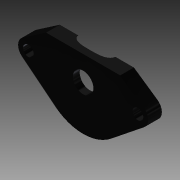
# Autodesk Inventor part: Bearing Cover
Saved by Autodesk Inventor 2013 (Build 170138000, 138)
## iProperties
Created: 2013-06-05
Part Number: Bearing Cover
Material: Generic
Document SubType Name: Modeling
Designer: mvarma
Density: 1 g/cm^3
Author: mvarma
Autodesk Inventor part; units mm, degrees
ref_plane "YZ Plane" through (0, 0, 0) normal (1, 0, 0) x (0, 1, 0)
ref_plane "XZ Plane" through (0, 0, 0) normal (0, 1, 0) x (-1, 0, 0)
ref_plane "XY Plane" through (0, 0, 0) normal (0, 0, 1) x (1, 0, 0)
sketch "Sketch1" plane through (0, 0, 0) normal (0, 0, 1) x (1, 0, 0)
  circle A0 centre (0, 0) radius 4.7625
  arc A1 (-17.1832, 11.43) -> (17.1832, 11.43) centre (0, 0) ccw
  arc A2 (-8.5725, 11.43) -> (8.5725, 11.43) centre (0, 0) ccw
  line L0 (-25.4, 0) -> (25.4, 0) construction
  circle A3 centre (-25.4, 0) radius 4.7625
  circle A4 centre (25.4, 0) radius 4.7625
  line L1 (-17.1832, 11.43) -> (17.1832, 11.43)
  arc A5 (8.5725, 11.43) -> (-8.5725, 11.43) centre (0, 0) ccw construction
  arc A6 (17.1832, 11.43) -> (-17.1832, 11.43) centre (0, 0) ccw construction
  line L2 (-17.1832, 11.43) -> (-28.0985, 3.9242)
  line L3 (17.1832, 11.43) -> (28.0985, 3.9242)
  line L4 (-28.3766, -3.7177) -> (-12.8984, -16.1101)
  line L5 (12.8984, -16.1101) -> (28.3766, -3.7177)
  arc A7 (-13.202, 11.43) -> (13.202, 11.43) centre (0, 0) ccw
  arc A8 (13.202, 11.43) -> (-13.202, 11.43) centre (0, 0) ccw construction
  dimension "d0" = 9.525
  dimension "d1" = 41.275
  dimension "d2" = 28.575
  dimension "d3" = 25.4
  dimension "d4" = 25.4
  dimension "d5" = 11.43
  dimension "d8" = 34.925
  dimension "d28" = 9.525
  constraints: 18 point on circle, 12 end point, 9 centre point, 8 tangent, 6 coincident, 4 point on line, 1 horizontal, 1 midpoint, 1 parallel
  measures "d0" diameter of A0
  measures "d1" diameter of A1
  measures "d2" diameter of A2
  measures "d3" distance of A2.centre L0.start
  measures "d4" distance of point (0, 0) L0.end
  measures "d5" distance between parallel lines of L0 L1
  measures "d8" diameter of A7
  measures "d28" diameter of A3
extrude "Extrusion4" add sketch "Sketch1" along normal blind 6.35
extrude "Extrusion5" cut sketch "Sketch1" along normal blind 3.175 contours L1 A2
hole "Hole1" at (-25.4, 0, 0) at (25.4, 0, 0) direction (0, 0, 1) diameter 4.9784 end through all clearance for "Socket Head Cap Screw" size "#10" standard "Ansi Unified Screw Threads"
fillet "Fillet2" radius 3.175 1 edges at (0, -14.2875, 3.175)
equation "\"d4\" = d3"
body "Solid1"
body "Solid2"
